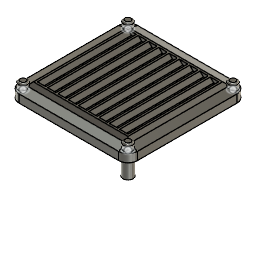
Prázdný modul (Autodesk Fusion 360 design; units mm, degrees)
Autodesk Fusion 360 part; units mm, degrees
note: some values were not read from the file. Chosen so that the rebuilt part matches the saved one: which pieces of a blend or face edit are solid. Set by a fixed rule: which sketch regions a step uses.
ref_plane "WorkPlane1" through (0, 0, -200) normal (0, 0, 1) x (1, 0, 0)
sketch "Sketch1" plane through (0, 0, 0) normal (0, 0, 1) x (1, 0, 0)
  line L0 (52.4, 52.4) -> (-52.4, 52.4) construction
  line L1 (-52.4, 52.4) -> (-52.4, -52.4) construction
  line L2 (-52.4, -52.4) -> (52.4, -52.4) construction
  line L3 (52.4, -52.4) -> (52.4, 52.4) construction
  line L4 (-52.4, -52.4) -> (52.4, 52.4) construction
  line L5 (-52.4, 52.4) -> (52.4, -52.4) construction
  line L6 (-43.9, 52.4) -> (43.9, 52.4)
  line L7 (52.4, -43.9) -> (52.4, 43.9)
  line L8 (43.9, -52.4) -> (-43.9, -52.4)
  line L9 (-52.4, 43.9) -> (-52.4, -43.9)
  arc A0 (-43.9, 52.4) -> (-52.4, 43.9) centre (-43.9, 43.9) ccw
  arc A1 (52.4, 43.9) -> (43.9, 52.4) centre (43.9, 43.9) ccw
  arc A2 (43.9, -52.4) -> (52.4, -43.9) centre (43.9, -43.9) ccw
  arc A3 (-52.4, -43.9) -> (-43.9, -52.4) centre (-43.9, -43.9) ccw
  circle A4 centre (-46.3749, 46.3749) radius 4
  line L10 (-49.2033, 49.2033) -> (-49.9104, 49.9104) construction
  circle A5 centre (46.3749, -46.3749) radius 4
  line L11 (-52.4, 0) -> (52.4, 0) construction
  circle A6 centre (-46.3749, -46.3749) radius 4
  circle A7 centre (46.3749, 46.3749) radius 4
  line L12 (41.7787, 41.7787) -> (-41.7787, 41.7787)
  line L13 (-41.7787, 41.7787) -> (-41.7787, -41.7787)
  line L14 (-41.7787, -41.7787) -> (41.7787, -41.7787)
  line L15 (41.7787, -41.7787) -> (41.7787, 41.7787)
  line L16 (41.7787, 41.7787) -> (-41.7787, -41.7787) construction
  line L17 (-41.7787, 41.7787) -> (41.7787, -41.7787) construction
  line L18 (41.7787, 41.7787) -> (43.5464, 43.5464) construction
  line L19 (40.0109, 40.0109) -> (-40.0109, 40.0109)
  line L20 (-40.0109, 40.0109) -> (-40.0109, -40.0109) construction
  line L21 (-40.0109, -40.0109) -> (40.0109, -40.0109)
  line L22 (40.0109, -40.0109) -> (40.0109, 40.0109) construction
  line L23 (40.0109, 40.0109) -> (-40.0109, -40.0109) construction
  line L24 (-40.0109, 40.0109) -> (40.0109, -40.0109) construction
  line L25 (40.0109, 40.0109) -> (41.7787, 41.7787) construction
  line L26 (-40.0109, 40.0109) -> (-41.7787, 40.0109) construction
  line L27 (-41.7787, 40.0109) -> (-41.7787, -40.0109) construction
  line L28 (-41.7787, -40.0109) -> (-40.0109, -40.0109) construction
  line L29 (-40.0109, -40.0109) -> (-40.0109, 40.0109)
  line L30 (-32.6909, -40.0109) -> (-30.9232, -40.0109)
  line L31 (-32.6909, 40.0109) -> (-32.6909, -40.0109)
  line L32 (-30.9232, -40.0109) -> (-30.9232, 40.0109)
  line L33 (-30.9232, 40.0109) -> (-32.6909, 40.0109)
  line L34 (-23.6032, -40.0109) -> (-21.8354, -40.0109)
  line L35 (-23.6032, 40.0109) -> (-23.6032, -40.0109)
  line L36 (-21.8354, -40.0109) -> (-21.8354, 40.0109)
  line L37 (-21.8354, 40.0109) -> (-23.6032, 40.0109)
  line L38 (-14.5155, -40.0109) -> (-12.7477, -40.0109)
  line L39 (-14.5155, 40.0109) -> (-14.5155, -40.0109)
  line L40 (-12.7477, -40.0109) -> (-12.7477, 40.0109)
  line L41 (-12.7477, 40.0109) -> (-14.5155, 40.0109)
  line L42 (-5.4277, -40.0109) -> (-3.66, -40.0109)
  line L43 (-5.4277, 40.0109) -> (-5.4277, -40.0109)
  line L44 (-3.66, -40.0109) -> (-3.66, 40.0109)
  line L45 (-3.66, 40.0109) -> (-5.4277, 40.0109)
  line L46 (3.66, -40.0109) -> (5.4278, -40.0109)
  line L47 (3.66, 40.0109) -> (3.66, -40.0109)
  line L48 (5.4278, -40.0109) -> (5.4278, 40.0109)
  line L49 (5.4278, 40.0109) -> (3.66, 40.0109)
  line L50 (12.7477, -40.0109) -> (14.5155, -40.0109)
  line L51 (12.7477, 40.0109) -> (12.7477, -40.0109)
  line L52 (14.5155, -40.0109) -> (14.5155, 40.0109)
  line L53 (14.5155, 40.0109) -> (12.7477, 40.0109)
  line L54 (21.8355, -40.0109) -> (23.6032, -40.0109)
  line L55 (21.8355, 40.0109) -> (21.8355, -40.0109)
  line L56 (23.6032, -40.0109) -> (23.6032, 40.0109)
  line L57 (23.6032, 40.0109) -> (21.8355, 40.0109)
  line L58 (30.9232, -40.0109) -> (32.691, -40.0109)
  line L59 (30.9232, 40.0109) -> (30.9232, -40.0109)
  line L60 (32.691, -40.0109) -> (32.691, 40.0109)
  line L61 (32.691, 40.0109) -> (30.9232, 40.0109)
  line L62 (40.0109, -40.0109) -> (41.7787, -40.0109)
  line L63 (40.0109, 40.0109) -> (40.0109, -40.0109)
  line L64 (41.7787, -40.0109) -> (41.7787, 40.0109) construction
  line L65 (41.7787, 40.0109) -> (40.0109, 40.0109) construction
  dimension "d4" = 104.8
  dimension "d6" = 8.5
  dimension "d7" = 8
  dimension "d8" = 1
  dimension "d9" = 2.5
  dimension "d10" = 2.5
  dimension "d13" = 81.7896
  dimension "d14" = 83.5574
  constraint horizontal L0
  constraint vertical L1
  constraint horizontal L2
  constraint vertical L3
  constraint coincident L4 origin
  constraint coincident L5 origin
  constraint equal L0 L3
  constraint coincident L0.end L9
  constraint coincident L0.end L6
  constraint tangent L9 A0
  constraint tangent L6 A0
  constraint coincident L0.start L6
  constraint coincident L0.start L7
  constraint tangent L6 A1
  constraint tangent L7 A1
  constraint equal A0 A1
  constraint coincident L2.end L7
  constraint coincident L2.end L8
  constraint tangent L7 A2
  constraint tangent L8 A2
  constraint equal A0 A2
  constraint coincident L1.end L8
  constraint coincident L1.end L9
  constraint tangent L8 A3
  constraint tangent L9 A3
  constraint equal A0 A3
  constraint coincident L5 A4.centre
  constraint coincident A4 L10.start
  constraint coincident L5 L10.start
  constraint midpoint A0 L10.end
  constraint symmetric L4 A4 A5
  constraint midpoint L9 L11.start
  constraint midpoint L7 L11.end
  constraint symmetric A4 L11 A6
  constraint symmetric A5 L11 A7
  constraint horizontal L12
  constraint perpendicular L12 L13
  constraint parallel L12 L14
  constraint parallel L13 L15
  constraint coincident L16 origin
  constraint coincident L17 origin
  constraint coincident L4 L12.start
  constraint coincident A7 L18.end
  constraint coincident L4 L18.end
  constraint horizontal L19
  constraint perpendicular L19 L20
  constraint parallel L19 L21
  constraint parallel L20 L22
  constraint coincident L23 origin
  constraint coincident L24 origin
  constraint coincident L4 L19.start
  constraint horizontal L26
  constraint vertical L27
  constraint horizontal L28
  constraint vertical L29
  constraint coincident L13 L27.end
  constraint collinear L21 L30
  measures "d4" distance of L0.start L0.end
  measures "d6" radius of A0
  measures "d7" diameter of A4
  measures "d8" distance of L10.start L10.end
  measures "d9" distance of L12.start L18.end
  measures "d10" distance of L12.start L19.start
extrude "Extrude1" add sketch "Sketch1" against normal blind 2 contours L6 L7 L8 L9 A0 A1 A2 A3 | A4 | A5 | A6 | A7 | L12 L13 L14 L15 | L19 L21 L60 L63 | L19 L21 L58 L59 L60 L61 | L19 L21 L56 L59 | L19 L21 L54 L55 L56 L57 | L19 L21 L52 L55 | L19 L21 L50 L51 L52 L53 | L19 L21 L48 L51 | L19 L21 L46 L47 L48 L49 | L19 L21 L44 L47 | L19 L21 L42 L43 L44 L45 | L19 L21 L40 L43 | L19 L21 L38 L39 L40 L41 | L19 L21 L36 L39 | L19 L21 L34 L35 L36 L37 | L19 L21 L32 L35 | L19 L21 L30 L31 L32 L33 | L19 L21 L29 L31 makes body 1
extrude "Extrude2" add sketch "Sketch1" along normal blind 3 contours L12 L13 L14 L15 | L19 L21 L58 L59 L60 L61 | L19 L21 L54 L55 L56 L57 | L19 L21 L50 L51 L52 L53 | L19 L21 L46 L47 L48 L49 | L19 L21 L42 L43 L44 L45 | L19 L21 L38 L39 L40 L41 | L19 L21 L34 L35 L36 L37 | L19 L21 L30 L31 L32 L33 bodies 1
chamfer "Chamfer1" distance 3 distance2 3 22 edges at (-40.0109, 0, 0) (-32.6909, 0, 0) (-30.9232, 0, 0) (-23.6032, 0, 0) (-21.8354, 0, 0) (-14.5155, 0, 0) (-12.7477, 0, 0) (-5.4277, 0, 0) (-3.66, 0, 0) (3.66, 0, 0) (5.4278, 0, 0) (12.7477, 0, 0) (14.5155, 0, 0) (21.8355, 0, 0) (23.6032, 0, 0) (30.9232, 0, 0) (32.691, 0, 0) (40.0109, 0, 0) (41.7787, 0, 0) (0, -41.7787, 0) (0, 41.7787, 0) (-41.7787, 0, 0) measured on face at (-35.1309, -13.337, 0) measured on face at (-35.1309, -13.337, 0) measured on face at (-28.4832, -13.337, 0) measured on face at (-28.4832, -13.337, 0) measured on face at (-16.9555, 13.337, 0) measured on face at (-16.9555, 13.337, 0) measured on face at (-7.8677, 13.337, 0) measured on face at (-7.8677, 13.337, 0) measured on face at (-1.22, 13.337, 0) measured on face at (-1.22, 13.337, 0) measured on face at (7.8677, -13.337, 0) measured on face at (7.8677, -13.337, 0) measured on face at (16.9555, 13.337, 0) measured on face at (16.9555, 13.337, 0) measured on face at (28.4832, -13.337, 0) measured on face at (28.4832, -13.337, 0) measured on face at (35.1309, 13.337, 0) measured on face at (35.1309, 13.337, 0) measured on face at (-48.8596, 13.9262, 0) measured on face at (-48.8596, 13.9262, 0) measured on face at (-48.8596, 13.9262, 0) measured on face at (-48.8596, 13.9262, 0) on bodies 1
extrude "Extrude4" add 1 faces at (-17.4667, -14.6333, -2) along direction (0, 0, -1) blind 2 on bodies 1 bodies 1
chamfer "Chamfer3" distance 2 distance2 7.6213 8 edges at (0, 52.4, 0) (49.9104, 49.9104, 0) (52.4, 0, 0) (49.9104, -49.9104, 0) (0, -52.4, 0) (-49.9104, -49.9104, 0) (-52.4, 0, 0) (-49.9104, 49.9104, 0) measured on face at (-14.6333, 52.4, -1.3333) measured on face at (-47.3187, -14.6333, 0) measured on face at (-47.3187, -14.6333, 0) measured on face at (-47.3187, -14.6333, 0) measured on face at (14.6333, -52.4, -1.3333) measured on face at (-47.3187, -14.6333, 0) measured on face at (-47.3187, -14.6333, 0) measured on face at (-47.3187, -14.6333, 0) on bodies 1
extrude "Extrude5" add 1 faces at (-17.4667, -14.6333, -4) along direction (0, 0, -1) blind 0.1 on bodies 1 bodies 1
sketch "Sketch2" plane through (0, 0, -4.1) normal (0, 0, -1) x (1, 0, 0)
  arc A0 (-52.4, -43.9) -> (-43.9, -52.4) centre (-43.9, -43.9) ccw
  line L0 (-43.9, -52.4) -> (43.9, -52.4)
  arc A1 (43.9, -52.4) -> (52.4, -43.9) centre (43.9, -43.9) ccw
  line L1 (52.4, -43.9) -> (52.4, 43.9)
  arc A2 (52.4, 43.9) -> (43.9, 52.4) centre (43.9, 43.9) ccw
  line L2 (43.9, 52.4) -> (-43.9, 52.4)
  arc A3 (-43.9, 52.4) -> (-52.4, 43.9) centre (-43.9, 43.9) ccw
  line L3 (-52.4, 43.9) -> (-52.4, -43.9)
  circle A4 centre (0, 0) radius 4.5
  arc A5 (50.4, 43.9) -> (43.9, 50.4) centre (43.9, 43.9) ccw
  line L4 (43.9, 50.4) -> (-43.9, 50.4)
  arc A6 (-43.9, 50.4) -> (-50.4, 43.9) centre (-43.9, 43.9) ccw
  line L5 (-50.4, 43.9) -> (-50.4, -43.9)
  arc A7 (-50.4, -43.9) -> (-43.9, -50.4) centre (-43.9, -43.9) ccw
  line L6 (-43.9, -50.4) -> (43.9, -50.4)
  arc A8 (43.9, -50.4) -> (50.4, -43.9) centre (43.9, -43.9) ccw
  line L7 (50.4, -43.9) -> (50.4, 43.9)
  dimension "d34" = 9
  dimension "d37" = -2
  measures "d34" diameter of A4
extrude "Extrude6" add sketch "Sketch2" along normal blind 64.9 contours A4 bodies 1
extrude "Extrude7" add sketch "Sketch2" along normal blind 5 contours A0 L0 A1 L1 A2 L2 A3 L3 bodies 1
chamfer "Chamfer4" distance 5 distance2 10 1 edges at (-4.1955, -1.6273, -4.1) measured on face at (0.1121, -35.0958, -4.1) on bodies 1
sketch "Sketch5" plane through (0, 0, -69) normal (0, 0, -1) x (1, 0, 0)
  circle A0 centre (0, 0) radius 4.5
  circle A1 centre (0, 0) radius 1.25
  dimension "d44" = 2.5
  constraint concentric A0 A1
  measures "d44" diameter of A1
extrude "Extrude8" cut sketch "Sketch5" against normal blind 17 contours A1 bodies 1
extrude "Extrude9" cut sketch "Sketch1" along normal blind -3 and the other way blind -5 contours A4 | A5 | A6 | A7 bodies 1
copy_body "Body->Comp1" bodies 1 removing the originals makes body 2 in component "Component'"
sketch "Sketch1 (2)" plane through (0, 0, -3) normal (0, 0, 1) x (-1, 0, 0) in component "Component''"
  circle A0 centre (-46.3749, 46.3749) radius 4
  circle A1 centre (-46.3749, 46.3749) radius 3.925
  circle A2 centre (-46.3749, 46.3749) radius 2.075
  dimension "d51" = 7.85
  dimension "d59" = 4.15
  constraint concentric A0 A1
  constraint concentric A0 A2
  measures "d51" diameter of A1
  measures "d59" diameter of A2
extrude "Extrude1'" add sketch "Sketch1 (2)" along normal blind 7.3 separate body contours A1 | A2 makes body 3 in component "Component''"
extrude "Extrude2'" cut sketch "Sketch1 (2)" along normal blind 3.2 contours A2 bodies 3 in component "Component''"
fillet "Fillet1" radius 1.5 1 edges at (50.0343, -44.9555, 4.3) on bodies 3 in component "Component''"
sketch "Sketch6" plane through (0, 0, -3) normal (0, 0, 1) x (-1, 0, 0)
  circle A0 centre (-46.3749, 46.3749) radius 4
  circle A1 centre (-46.3749, 46.3749) radius 2
  line L0 (0, -2.5) -> (0, -20)
  circle A2 centre (46.3749, 46.3749) radius 2
  line L1 (-20, 0) -> (-2.5, 0)
  circle A3 centre (46.3749, -46.3749) radius 2
  circle A4 centre (-46.3749, -46.3749) radius 2
  dimension "d56" = 4
  constraint concentric A0 A1
  constraint symmetric A1 L0 A2
  constraint symmetric A1 L1 A4
  constraint symmetric A2 L1 A3
  measures "d56" diameter of A1
extrude "Extrude1''" add sketch "Sketch6" along normal blind 3 contours A1 | A2 | A3 | A4 bodies 2 in component "Component'"
component "Component'" placed x (1, 0, 0) y (0, 1, 0) z (0, 0, 1) at (0, 0, 0)
component "Component''" placed x (1, 0, 0) y (0, 1, 0) z (0, 0, 1) at (0, 0, 0)
component "Component''" placed x (1, 0, 0) y (0, 1, 0) z (0, 0, 1) at (0, 92.7497, 0)
component "Component''" placed x (1, 0, 0) y (0, 1, 0) z (0, 0, 1) at (-92.7497, 0, 0)
component "Component''" placed x (1, 0, 0) y (0, 1, 0) z (0, 0, 1) at (-92.7497, 92.7497, 0)
equation "d35 = 67 mm - 2.10 mm"
equation "d51 = 8 mm - 0.15 mm"
equation "d52 = 1.3 mm + 6 mm"
